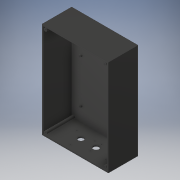
# Autodesk Inventor part: base da caixa
Saved by Autodesk Inventor 2019.4 (Build 234330000, 330)
## iProperties
Created: 2020-11-09
Part Number: base da caixa
Material: Plástico PC/ABS
Document SubType Name: Modeling
Designer: Lattes
Density: 0.357273 g/cm^3
Appearance: Liso - Preto
Author: Lattes
Autodesk Inventor part; units mm, degrees
ref_plane "YZ Plane" through (0, 0, 0) normal (1, 0, 0) x (0, 1, 0)
ref_plane "XZ Plane" through (0, 0, 0) normal (0, 1, 0) x (-1, 0, 0)
ref_plane "XY Plane" through (0, 0, 0) normal (0, 0, 1) x (1, 0, 0)
sketch "Esboço1" plane through (0, 0, 0) normal (0, 0, 1) x (1, 0, 0)
  line L0 (0, 0) -> (185, 0)
  line L1 (185, 0) -> (185, 265)
  line L2 (185, 265) -> (0, 265)
  line L3 (0, 265) -> (0, 0)
  line L4 (0, 0) -> (12, 0)
  line L5 (12, 0) -> (12, 12)
  line L6 (185, 0) -> (173, 0)
  line L7 (173, 0) -> (173, 12)
  line L8 (0, 265) -> (0, 253)
  line L9 (0, 253) -> (12, 253)
  line L10 (185, 265) -> (185, 253)
  line L11 (185, 253) -> (173, 253)
  circle A0 centre (173, 253) radius 4
  circle A1 centre (12, 253) radius 4
  circle A2 centre (12, 12) radius 4
  circle A3 centre (173, 12) radius 4
  line L12 (180, 5) -> (180, 260)
  line L13 (180, 260) -> (5, 260)
  line L14 (5, 260) -> (180, 260)
  line L15 (180, 260) -> (180, 5)
  line L16 (180, 5) -> (5, 5)
  line L17 (5, 5) -> (5, 260)
  dimension "d2" = 185
  dimension "d3" = 265
  dimension "d4" = 12
  dimension "d5" = 12
  dimension "d6" = 12
  dimension "d7" = 12
  dimension "d8" = 12
  dimension "d9" = 12
  dimension "d10" = 12
  dimension "d11" = 12
  dimension "d12" = 8
  dimension "d13" = 8
  dimension "d14" = 8
  dimension "d15" = 8
  dimension "d18" = 255
  dimension "d19" = 175
  constraints: 36 end point, 9 perpendicular, 4 centre point, 4 coincident, 4 point on line, 2 horizontal, 2 parallel
  measures "d2" distance of L0.start L0.end
  measures "d3" distance of L0.end L1.end
  measures "d4" distance of L0.start L4.end
  measures "d5" distance of L4.end L5.end
  measures "d6" distance of L0.end L6.end
  measures "d7" distance of L6.end L7.end
  measures "d8" distance of L2.end L8.end
  measures "d9" distance of L8.end L9.end
  measures "d10" distance of L1.end L10.end
  measures "d11" distance of L10.end L11.end
  measures "d12" diameter of A0
  measures "d13" diameter of A1
  measures "d14" diameter of A2
  measures "d15" diameter of A3
  measures "d18" distance of L12.start L12.end
  measures "d19" distance of L12.end L13.end
sketch "Esboço2" plane through (0, 0, 0) normal (0, 0, 1) x (1, 0, 0)
  line L0 (185, 265) -> (185, 253)
  line L1 (180, 5) -> (180, 260)
  line L2 (180, 260) -> (5, 260)
  line L3 (5, 260) -> (180, 260)
  line L4 (180, 260) -> (180, 5)
  line L5 (180, 5) -> (5, 5)
  line L6 (5, 5) -> (5, 260)
  point P0 (0, 0)
  dimension "d34" = 255
  dimension "d35" = 175
  constraints: 14 end point, 2 parallel, 2 perpendicular, 1 horizontal
  measures "d34" distance of L1.start L1.end
  measures "d35" distance of L1.end L2.end
extrude "Extrusão1" add sketch "Esboço2" along normal blind 3
sketch "Esboço3" plane through (0, 0, 3) normal (0, 0, 1) x (1, 0, 0)
  circle A0 centre (173, 253) radius 4
  circle A1 centre (12, 253) radius 4
  circle A2 centre (12, 12) radius 4
  circle A3 centre (173, 12) radius 4
  line L0 (180, 5) -> (180, 260)
  line L1 (180, 260) -> (5, 260)
  line L2 (5, 260) -> (180, 260)
  line L3 (180, 260) -> (180, 5)
  line L4 (180, 5) -> (5, 5)
  line L5 (5, 5) -> (5, 260)
  circle A4 centre (12, 12) radius 1.575
  circle A5 centre (12, 253) radius 1.575
  circle A6 centre (173, 253) radius 1.575
  circle A7 centre (173, 12) radius 1.575
  line L6 (173, 12) -> (173, 11)
  dimension "d48" = 8
  dimension "d49" = 8
  dimension "d50" = 8
  dimension "d51" = 8
  dimension "d52" = 255
  dimension "d53" = 175
  dimension "d54" = 3.15
  dimension "d55" = 3.15
  dimension "d56" = 3.15
  dimension "d57" = 3.15
  dimension "d219" = 1
  constraints: 14 end point, 8 centre point, 4 coincident, 2 parallel, 2 perpendicular, 1 horizontal, 1 vertical
  measures "d48" diameter of A0
  measures "d49" diameter of A1
  measures "d50" diameter of A2
  measures "d51" diameter of A3
  measures "d52" distance of L0.start L0.end
  measures "d53" distance of L0.end L1.end
  measures "d54" diameter of A4
  measures "d55" diameter of A5
  measures "d56" diameter of A6
  measures "d57" diameter of A7
  measures "d219" distance of L6.start L6.end
extrude "Extrusão2" add sketch "Esboço3" along normal blind 77 contours A0 | A1 | A2 | A3
sketch "Esboço4" plane through (0, 0, 3) normal (0, 0, 1) x (1, 0, 0)
  line L0 (0, 0) -> (185, 0)
  line L1 (185, 0) -> (185, 265)
  line L2 (185, 265) -> (0, 265)
  line L3 (0, 265) -> (0, 0)
  line L4 (0, 0) -> (12, 0)
  line L5 (185, 0) -> (173, 0)
  line L6 (0, 265) -> (0, 253)
  line L7 (185, 265) -> (185, 253)
  line L8 (0, 265) -> (0, 220)
  line L9 (0, 220) -> (32.5, 220)
  line L10 (0, 220) -> (0, 168)
  line L11 (0, 168) -> (32.5, 168)
  line L12 (92.5, 265) -> (92.5, 240)
  line L13 (0, 0) -> (0, 45)
  line L14 (0, 45) -> (32.5, 45)
  line L15 (185, 0) -> (185, 45)
  line L16 (185, 45) -> (152.5, 45)
  circle A0 centre (92.5, 240) radius 3
  circle A1 centre (92.5, 240) radius 1.5
  circle A2 centre (32.5, 220) radius 1.5
  circle A3 centre (32.5, 220) radius 3
  circle A4 centre (32.5, 168) radius 1.5
  circle A5 centre (32.5, 168) radius 3
  circle A6 centre (32.5, 45) radius 1.5
  circle A7 centre (32.5, 45) radius 3
  circle A8 centre (152.5, 45) radius 1.5
  circle A9 centre (152.5, 45) radius 3
  line L17 (185, 265) -> (185, 220)
  line L18 (185, 220) -> (152.5, 220)
  line L19 (185, 220) -> (185, 168)
  line L20 (185, 168) -> (152.5, 168)
  circle A10 centre (152.5, 168) radius 1.5
  circle A11 centre (152.5, 168) radius 3
  circle A12 centre (152.5, 220) radius 1.5
  circle A13 centre (152.5, 220) radius 3
  point P0 (180, 5)
  point P1 (5, 260)
  dimension "d60" = 185
  dimension "d61" = 265
  dimension "d64" = 12
  dimension "d66" = 12
  dimension "d76" = 45
  dimension "d77" = 32.5
  dimension "d78" = 52
  dimension "d79" = 32.5
  dimension "d84" = 25
  dimension "d85" = 45
  dimension "d86" = 32.5
  dimension "d88" = 32.5
  dimension "d89" = 6
  dimension "d90" = 3
  dimension "d91" = 3
  dimension "d92" = 6
  dimension "d93" = 3
  dimension "d94" = 6
  dimension "d99" = 3
  dimension "d100" = 6
  dimension "d101" = 3
  dimension "d102" = 6
  dimension "d149" = 32.5
  dimension "d150" = 52
  dimension "d151" = 32.5
  dimension "d152" = 3
  dimension "d153" = 6
  dimension "d154" = 3
  dimension "d155" = 6
  constraints: 42 end point, 14 centre point, 14 coincident, 10 point on line, 9 perpendicular, 1 horizontal, 1 midpoint, 1 vertical
  measures "d60" distance of L0.start L0.end
  measures "d61" distance of L0.end L1.end
  measures "d64" distance of L0.end L5.end
  measures "d66" distance of L2.end L6.end
  measures "d76" distance of L2.end L8.end
  measures "d77" distance of L8.end L9.end
  measures "d78" distance of L8.end L10.end
  measures "d79" distance of L10.end L11.end
  measures "d84" distance of L12.start L12.end
  measures "d85" distance of L0.start L13.end
  measures "d86" distance of L13.end L14.end
  measures "d88" distance of L15.end L16.end
  measures "d89" diameter of A0
  measures "d90" diameter of A1
  measures "d91" diameter of A2
  measures "d92" diameter of A3
  measures "d93" diameter of A4
  measures "d94" diameter of A5
  measures "d99" diameter of A6
  measures "d100" diameter of A7
  measures "d101" diameter of A8
  measures "d102" diameter of A9
  measures "d149" distance of L17.end L18.end
  measures "d150" distance of L17.end L19.end
  measures "d151" distance of L19.end L20.end
  measures "d152" diameter of A10
  measures "d153" diameter of A11
  measures "d154" diameter of A12
  measures "d155" diameter of A13
sketch "Esboço5" plane through (0, 0, 3) normal (0, 0, 1) x (1, 0, 0)
  circle A0 centre (92.5, 240) radius 3
  circle A1 centre (92.5, 240) radius 1.5
  circle A2 centre (32.5, 220) radius 1.5
  circle A3 centre (32.5, 220) radius 3
  circle A4 centre (32.5, 168) radius 1.5
  circle A5 centre (32.5, 168) radius 3
  circle A6 centre (147.5, 215) radius 1.5
  circle A7 centre (147.5, 215) radius 3
  circle A8 centre (147.5, 163) radius 1.5
  circle A9 centre (147.5, 163) radius 3
  circle A10 centre (32.5, 45) radius 1.5
  circle A11 centre (32.5, 45) radius 3
  circle A12 centre (152.5, 45) radius 1.5
  circle A13 centre (152.5, 45) radius 3
  dimension "d132" = 6
  dimension "d133" = 3
  dimension "d134" = 3
  dimension "d135" = 6
  dimension "d136" = 3
  dimension "d137" = 6
  dimension "d138" = 3
  dimension "d139" = 6
  dimension "d142" = 3
  dimension "d143" = 6
  dimension "d144" = 3
  dimension "d145" = 6
  dimension "d146" = 6
  dimension "d147" = 3
  constraints: 14 centre point, 7 coincident
  measures "d132" diameter of A0
  measures "d133" diameter of A1
  measures "d134" diameter of A2
  measures "d135" diameter of A3
  measures "d136" diameter of A4
  measures "d137" diameter of A5
  measures "d138" diameter of A6
  measures "d139" diameter of A7
  measures "d142" diameter of A10
  measures "d143" diameter of A11
  measures "d144" diameter of A12
  measures "d145" diameter of A13
  measures "d146" diameter of A9
  measures "d147" diameter of A8
sketch "Esboço7" plane through (0, 0, 3) normal (0, 0, 1) x (1, 0, 0)
  line L0 (0, 0) -> (185, 0)
  line L1 (185, 0) -> (185, 265)
  line L2 (185, 265) -> (0, 265)
  line L3 (0, 265) -> (0, 0)
  line L4 (0, 0) -> (12, 0)
  line L5 (12, 0) -> (12, 12)
  line L6 (185, 0) -> (173, 0)
  line L7 (173, 0) -> (173, 12)
  line L8 (0, 265) -> (0, 253)
  line L9 (0, 253) -> (12, 253)
  line L10 (185, 265) -> (185, 253)
  line L11 (185, 253) -> (173, 253)
  circle A0 centre (173, 253) radius 4
  circle A1 centre (12, 253) radius 4
  circle A2 centre (12, 12) radius 4
  circle A3 centre (173, 12) radius 4
  line L12 (180, 5) -> (180, 260)
  line L13 (180, 260) -> (5, 260)
  line L14 (5, 260) -> (180, 260)
  line L15 (180, 260) -> (180, 5)
  line L16 (180, 5) -> (5, 5)
  line L17 (5, 5) -> (5, 260)
  line L18 (5, 5) -> (180, 5) projected
  line L19 (5, 5) -> (0, 5)
  dimension "d187" = 185
  dimension "d188" = 265
  dimension "d189" = 12
  dimension "d190" = 12
  dimension "d191" = 12
  dimension "d192" = 12
  dimension "d193" = 12
  dimension "d194" = 12
  dimension "d195" = 12
  dimension "d196" = 12
  dimension "d197" = 8
  dimension "d198" = 8
  dimension "d199" = 8
  dimension "d200" = 8
  dimension "d201" = 255
  dimension "d202" = 175
  constraints: 38 end point, 10 perpendicular, 5 point on line, 4 centre point, 4 coincident, 2 horizontal, 2 parallel
  measures "d187" distance of L0.start L0.end
  measures "d188" distance of L0.end L1.end
  measures "d189" distance of L0.start L4.end
  measures "d190" distance of L4.end L5.end
  measures "d191" distance of L0.end L6.end
  measures "d192" distance of L6.end L7.end
  measures "d193" distance of L2.end L8.end
  measures "d194" distance of L8.end L9.end
  measures "d195" distance of L1.end L10.end
  measures "d196" distance of L10.end L11.end
  measures "d197" diameter of A0
  measures "d198" diameter of A1
  measures "d199" diameter of A2
  measures "d200" diameter of A3
  measures "d201" distance of L12.start L12.end
  measures "d202" distance of L12.end L13.end
sketch "Esboço8" plane through (0, 0, 3) normal (0, 0, 1) x (1, 0, 0)
  line L0 (5, 5) -> (180, 5) projected
  line L1 (92.5, 5) -> (179, 5)
  line L2 (5, 260) -> (5, 5) projected
  line L3 (180, 260) -> (5, 260) projected
  line L4 (179, 6) -> (179, 259)
  line L5 (179, 259) -> (6, 259)
  line L6 (6, 259) -> (6, 6)
  line L7 (6, 6) -> (179, 6)
  line L8 (179, 6) -> (179, 259)
  line L9 (6, 6) -> (6, 3)
  line L10 (6, 3) -> (3, 3)
  line L11 (179, 259) -> (179, 262)
  line L12 (179, 262) -> (182, 262)
  line L13 (182, 262) -> (3, 262)
  line L14 (3, 262) -> (3, 3)
  line L15 (3, 3) -> (182, 3)
  line L16 (182, 3) -> (182, 262)
  point P0 (0, 0)
  dimension "d207" = 86.5
  dimension "d211" = 3
  dimension "d212" = 3
  dimension "d213" = 3
  dimension "d214" = 3
  constraints: 28 end point, 4 parallel, 4 perpendicular, 2 horizontal, 1 midpoint, 1 point on line, 1 vertical
  measures "d207" distance of L1.start L1.end
  measures "d211" distance of L6.end L9.end
  measures "d212" distance of L9.end L10.end
  measures "d213" distance of L4.end L11.end
  measures "d214" distance of L11.end L12.end
extrude "Extrusão4" add sketch "Esboço8" along normal blind 77 and the other way blind 3 contours L2 L3 L11 L5 L6 L9 L0 | L0 L9 L10 L14 L13 L11 L3 L2 | L9 L7 L4 L11 L12 L16 L15
sketch "Esboço9" plane through (0, 0, 3) normal (0, 0, 1) x (1, 0, 0)
  point P0 (0, 0)
sketch "Esboço6" plane through (0, 0, 3) normal (0, 0, 1) x (1, 0, 0)
  line L0 (92.5, 265) -> (92.5, 240)
  circle A0 centre (92.5, 240) radius 3
  circle A1 centre (92.5, 240) radius 1.5
  circle A2 centre (32.5, 220) radius 1.5
  circle A3 centre (32.5, 220) radius 3
  circle A4 centre (152.5, 220) radius 1.5
  circle A5 centre (152.5, 220) radius 3
  line L1 (180, 5) -> (180, 8)
  line L2 (180, 5) -> (180, 260) projected
  line L3 (180, 8) -> (180, 16)
  circle A6 centre (173, 12) radius 1.575 projected
  line L4 (6, 6) -> (179, 6) projected
  line L5 (179, 6) -> (179, 47)
  line L6 (179, 259) -> (179, 6) projected
  circle A7 centre (152.5, 47) radius 1.5
  circle A8 centre (152.5, 47) radius 3
  line L7 (6, 6) -> (6, 47)
  line L8 (6, 6) -> (6, 259) projected
  circle A9 centre (32.5, 47) radius 1.5
  circle A10 centre (32.5, 47) radius 3
  line L9 (32.5, 47) -> (32.5, 165)
  circle A11 centre (32.5, 165) radius 1.5
  circle A12 centre (32.5, 165) radius 3
  line L10 (152.5, 47) -> (152.5, 165)
  circle A13 centre (152.5, 165) radius 1.5
  circle A14 centre (152.5, 165) radius 3
  dimension "d164" = 25
  dimension "d168" = 6
  dimension "d169" = 3
  dimension "d170" = 3
  dimension "d171" = 6
  dimension "d183" = 3
  dimension "d184" = 6
  dimension "d203" = 3
  dimension "d204" = 8
  dimension "d220" = 41
  dimension "d222" = 3
  dimension "d223" = 6
  dimension "d224" = 41
  dimension "d227" = 3
  dimension "d228" = 6
  dimension "d240" = 118
  dimension "d241" = 3
  dimension "d242" = 6
  dimension "d243" = 118
  dimension "d244" = 3
  dimension "d245" = 6
  constraints: 14 centre point, 14 end point, 10 coincident, 4 point on line, 1 vertical
  measures "d164" distance of L0.start L0.end
  measures "d168" diameter of A0
  measures "d169" diameter of A1
  measures "d170" diameter of A2
  measures "d171" diameter of A3
  measures "d183" diameter of A4
  measures "d184" diameter of A5
  measures "d203" distance of L1.start L1.end
  measures "d204" distance of L1.end L3.end
  measures "d220" distance of L4.end L5.end
  measures "d222" diameter of A7
  measures "d223" diameter of A8
  measures "d224" distance of L4.start L7.end
  measures "d227" diameter of A9
  measures "d228" diameter of A10
  measures "d240" distance of L9.start L9.end
  measures "d241" diameter of A11
  measures "d242" diameter of A12
  measures "d243" distance of L10.start L10.end
  measures "d244" diameter of A13
  measures "d245" diameter of A14
extrude "Extrusão6" add sketch "Esboço6" along normal blind 5 contours A8 | A14 | A10 | A12
sketch "posição dos furos" plane through (0, 0, 3) normal (0, 0, 1) x (1, 0, 0)
  line L0 (179, 6) -> (179, 53.5)
  line L1 (179, 6) -> (179, 259)
  line L2 (179, 53.5) -> (179, 47)
  line L3 (179, 47) -> (142.8647, 47)
  circle A0 centre (152.5, 47) radius 1.5
  line L4 (152.5, 47) -> (152.5, 6)
  circle A1 centre (152.5, 47) radius 3
  line L5 (152.5, 50) -> (152.5, 53)
  line L6 (152.5, 53) -> (179, 53)
  circle A2 centre (152.5, 47) radius 6
  line L7 (152.5, 47) -> (164, 47)
  line L8 (152.5, 41) -> (164, 41)
  line L9 (164, 7) -> (167, 7)
  line L10 (164, 7) -> (164, 41)
  line L11 (167, 7) -> (167, 17.182)
  line L12 (167, 17.182) -> (178, 17.182)
  line L13 (178, 17.182) -> (178, 53)
  circle A3 centre (32.5, 47) radius 1.5
  line L14 (32.5, 47) -> (32.5, 165)
  circle A4 centre (173, 12) radius 1.575 projected
  circle A5 centre (173, 12) radius 1.575
  circle A6 centre (173, 12) radius 3.9962
  point P0 (0, 0)
  point P1 (0, 0)
  dimension "d248" = 47.5
  dimension "d249" = 6.5
  dimension "d250" = 3
  dimension "d251" = 11.5
  dimension "d252" = 10.182
  dimension "d253" = 11
  dimension "d254" = 118
  constraints: 30 end point, 6 point on line, 5 centre point, 4 perpendicular, 4 vertical, 3 coincident, 2 point on circle, 1 tangent, 1 vertical alignment, 2 other
  measures "d248" distance of L0.start L0.end
  measures "d249" distance of L0.end L2.end
  measures "d250" distance of L5.start L5.end
  measures "d251" distance of L7.start L7.end
  measures "d252" distance of L9.end L11.end
  measures "d253" distance of L11.end L12.end
  measures "d254" distance of L14.start L14.end
sketch "furos 5mm caixa" plane through (0, 0, 3) normal (0, 0, 1) x (1, 0, 0)
  line L0 (92.5, 265) -> (92.5, 240)
  circle A0 centre (92.5, 240) radius 3
  circle A1 centre (92.5, 240) radius 1.5
  circle A2 centre (32.5, 220) radius 1.5
  circle A3 centre (32.5, 220) radius 3
  circle A4 centre (152.5, 220) radius 1.5
  circle A5 centre (152.5, 220) radius 3
  line L1 (180, 5) -> (180, 8)
  line L2 (180, 5) -> (180, 260)
  line L3 (180, 8) -> (180, 16)
  circle A6 centre (173, 12) radius 1.575
  line L4 (6, 6) -> (179, 6)
  line L5 (179, 6) -> (179, 47)
  line L6 (179, 259) -> (179, 6)
  circle A7 centre (152.5, 47) radius 1.5
  circle A8 centre (152.5, 47) radius 3
  line L7 (6, 6) -> (6, 47)
  line L8 (6, 6) -> (6, 259)
  circle A9 centre (32.5, 47) radius 1.5
  circle A10 centre (32.5, 47) radius 3
  line L9 (32.5, 47) -> (32.5, 165)
  circle A11 centre (32.5, 165) radius 1.5
  circle A12 centre (32.5, 165) radius 3
  line L10 (152.5, 47) -> (152.5, 165)
  circle A13 centre (152.5, 165) radius 1.5
  circle A14 centre (152.5, 165) radius 3
  point P0 (0, 0)
  dimension "d255" = 25
  dimension "d256" = 6
  dimension "d257" = 3
  dimension "d258" = 3
  dimension "d259" = 6
  dimension "d260" = 3
  dimension "d261" = 6
  dimension "d262" = 3
  dimension "d263" = 8
  dimension "d264" = 41
  dimension "d265" = 3
  dimension "d266" = 6
  dimension "d267" = 41
  dimension "d268" = 3
  dimension "d269" = 6
  dimension "d270" = 118
  dimension "d271" = 3
  dimension "d272" = 6
  dimension "d273" = 118
  dimension "d274" = 3
  dimension "d275" = 6
  constraints: 22 end point, 15 centre point, 10 coincident, 4 point on line, 1 vertical
  measures "d255" distance of L0.start L0.end
  measures "d256" diameter of A0
  measures "d257" diameter of A1
  measures "d258" diameter of A2
  measures "d259" diameter of A3
  measures "d260" diameter of A4
  measures "d261" diameter of A5
  measures "d262" distance of L1.start L1.end
  measures "d263" distance of L1.end L3.end
  measures "d264" distance of L4.end L5.end
  measures "d265" diameter of A7
  measures "d266" diameter of A8
  measures "d267" distance of L4.start L7.end
  measures "d268" diameter of A9
  measures "d269" diameter of A10
  measures "d270" distance of L9.start L9.end
  measures "d271" diameter of A11
  measures "d272" diameter of A12
  measures "d273" distance of L10.start L10.end
  measures "d274" diameter of A13
  measures "d275" diameter of A14
sketch "Esboço13" plane through (3, 3, 80) normal (0, -1, 0) x (1, 0, 0)
  circle A0 centre (65, -40) radius 7.5
  point P0 (-3, -80)
  point P1 (0, -80)
  dimension "d279" = 15
  constraints: 1 centre point
  measures "d279" diameter of A0
extrude "Extrusão7" cut sketch "Esboço13" against normal blind 10
sketch "Esboço14" plane through (6, 6, 3) normal (0, 1, 0) x (1, 0, 0)
  point P0 (-6, 3)
sketch "Esboço15" plane through (3, 3, 80) normal (0, -1, 0) x (1, 0, 0)
  circle A0 centre (65, -12) radius 1.5
  point P0 (-3, -80)
  dimension "d283" = 3
  constraints: 1 centre point
  measures "d283" diameter of A0
extrude "Extrusão8" cut sketch "Esboço15" against normal blind 10
pattern_circular "Padrão circular1" count 3 over 360 about axis through (68, 3, 40) along (0, 1, 0) of "Extrusão8"
sketch "Esboço16" plane through (3, 3, 80) normal (0, -1, 0) x (1, 0, 0)
  point P0 (-3, -80)
sketch "Esboço17" plane through (3, 3, 80) normal (0, -1, 0) x (1, 0, 0)
  line L0 (179, -80) -> (164, -80)
  line L1 (179, -80) -> (98, -80)
  line L2 (0, -80) -> (179, -80) projected
  line L3 (3, 0) -> (176, 0) projected
  line L4 (98, 0) -> (98, -80)
  line L5 (164, 0) -> (164, -80)
  circle A0 centre (106, -40) radius 8
  circle A1 centre (148, -40) radius 8
  point P0 (-3, -80)
  dimension "d289" = 15
  dimension "d290" = 81
  dimension "d306" = 16
  constraints: 8 end point, 3 point on line, 2 centre point, 2 perpendicular, 1 horizontal
  measures "d289" distance of L0.start L0.end
  measures "d290" distance of L0.start L1.end
  measures "d306" diameter of A1
extrude "Extrusão11" cut sketch "Esboço17" against normal blind 10 contours A0 | A1
sketch "Esboço19" plane through (3, 3, 80) normal (0, -1, 0) x (1, 0, 0)
  circle A0 centre (148, -40) radius 8 projected
  line L0 (148, -40) -> (148, -24.575)
  line L1 (148, -40) -> (148, -55.425)
  circle A1 centre (148, -55.425) radius 1.5
  circle A2 centre (148, -24.575) radius 1.5
  circle A3 centre (106, -40) radius 8 projected
  line L2 (106, -40) -> (106, -24.575)
  line L3 (106, -40) -> (106, -55.425)
  circle A4 centre (106, -55.425) radius 1.5
  circle A5 centre (106, -24.575) radius 1.5
  point P0 (-3, -80)
  dimension "d309" = 15.425
  dimension "d310" = 15.425
  dimension "d311" = 3
  dimension "d312" = 3
  dimension "d313" = 15.425
  dimension "d314" = 15.425
  dimension "d315" = 3
  dimension "d316" = 3
  constraints: 8 end point, 4 centre point, 4 coincident, 4 vertical
  measures "d309" distance of L0.start L0.end
  measures "d310" distance of L0.start L1.end
  measures "d311" diameter of A1
  measures "d312" diameter of A2
  measures "d313" distance of L2.start L2.end
  measures "d314" distance of L2.start L3.end
  measures "d315" diameter of A4
  measures "d316" diameter of A5
extrude "Extrusão12" cut sketch "Esboço19" against normal blind 10 contours A1 | A2 | A4 | A5
sketch "Esboço20" plane through (0, 0, 0) normal (0, 0, -1) x (-1, 0, 0)
  line L0 (-182, 3) -> (-3, 3) projected
  circle A0 centre (-112.5, 247) radius 3.5
  circle A1 centre (-72.5, 247) radius 3.5
  point P0 (0, 0)
  dimension "d339" = 7
  dimension "d340" = 7
  constraints: 2 centre point
  measures "d339" diameter of A0
  measures "d340" diameter of A1
extrude "Extrusão15" cut sketch "Esboço20" against normal blind 10
sketch "Esboço21" plane through (0, 0, 3) normal (0, 0, 1) x (1, 0, 0)
  line L0 (6, 259) -> (179, 259) projected
  line L1 (92.5, 259) -> (92.5, 236)
  line L2 (92.5, 236) -> (92.5, 242)
  circle A0 centre (92.5, 239) radius 3
  circle A1 centre (92.5, 239) radius 1.5
  line L3 (92.5, 220) -> (92.5, 215)
  line L4 (92.5, 239) -> (92.5, 217)
  line L5 (92.5, 217) -> (152.5, 217)
  circle A2 centre (152.5, 217) radius 1.5
  circle A3 centre (152.5, 217) radius 3
  circle A4 centre (32.5, 217) radius 1.5
  circle A5 centre (32.5, 217) radius 3
  point P0 (0, 0)
  dimension "d349" = 23
  dimension "d350" = 6
  dimension "d351" = 3
  dimension "d352" = 19
  dimension "d353" = 5
  dimension "d355" = 22
  dimension "d356" = 60
  dimension "d357" = 3
  dimension "d358" = 6
  constraints: 10 end point, 5 centre point, 4 coincident, 2 midpoint, 2 symmetric about line, 2 vertical, 1 perpendicular, 1 point on line, 1 vertical alignment, 4 other
  measures "d349" distance of L1.start L1.end
  measures "d350" distance of L1.end L2.end
  measures "d351" diameter of A1
  measures "d352" distance of L4.start L3.start
  measures "d353" distance of L3.start L3.end
  measures "d355" distance of L4.start L4.end
  measures "d356" distance of L4.end L5.end
  measures "d357" diameter of A2
  measures "d358" diameter of A3
extrude "Extrusão16" add sketch "Esboço21" along normal blind 5 contours A0 L1 A1 | A3 | L1 A1 A0 | A5
sketch "Esboço22" plane through (0, 0, 80) normal (0, 0, 1) x (1, 0, 0)
  line L0 (3, 3) -> (182, 3) projected
  line L1 (3, 262) -> (182, 262)
  line L2 (182, 262) -> (182, 3)
  line L3 (182, 3) -> (3, 3)
  line L4 (3, 3) -> (3, 262)
  line L5 (6, 6) -> (179, 6) projected
  line L6 (179, 259) -> (6, 259) projected
  line L7 (179, 6) -> (6, 6)
  line L8 (6, 6) -> (6, 259)
  line L9 (6, 259) -> (179, 259)
  line L10 (179, 259) -> (179, 6)
  point P0 (0, 0)
  constraints: 16 end point, 4 parallel, 2 horizontal, 2 perpendicular
